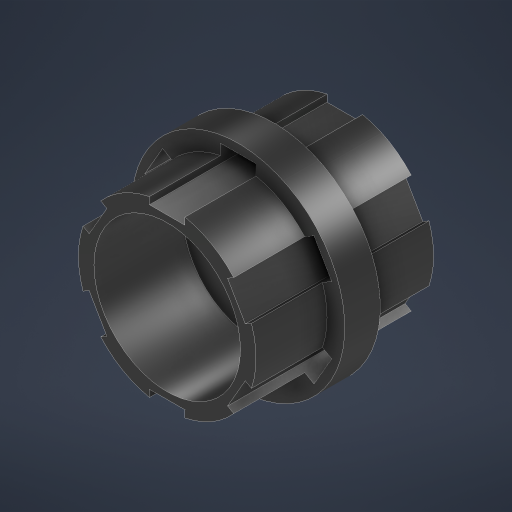
# Autodesk Inventor part: koło
Saved by Autodesk Inventor 2023.4 (Build 274418000, 418)
## iProperties
Created: 2025-10-31
Part Number: koło
Material: Tworzywo sztuczne PET
Document SubType Name: Modeling
Designer: Jakub Borsukiewicz
Density: 1.541 g/cm^3
Appearance: Lśniąca — czarna
Author: Jakub Borsukiewicz
Autodesk Inventor part; units mm, degrees
ref_plane "YZ Plane" through (0, 0, 0) normal (1, 0, 0) x (0, 1, 0)
ref_plane "XZ Plane" through (0, 0, 0) normal (0, 1, 0) x (-1, 0, 0)
sketch "Szkic1" plane through (0, 0, 0) normal (0, 0, 1) x (1, 0, 0)
  line L0 (-14, 0) -> (14, 0) projected
  line L1 (0, -14) -> (0, 14) projected
  circle A0 centre (0, 0) radius 10
  circle A1 centre (0, 0) radius 1.8
  line L2 (-1.3416, 1.2) -> (1.3416, 1.2)
  dimension "d1" = 20
  dimension "d2" = 3.6
  dimension "d3" = 1.2
  constraints: 2 centre point, 2 coincident, 2 end point, 2 point on circle, 1 perpendicular
  measures "d1" diameter of A0
  measures "d2" diameter of A1
  measures "d3" distance between parallel lines of L0 L2
extrude "Wyciągnięcie proste1" add sketch "Szkic1" along normal blind 20 contours A1 L1 A0 L0 | L0 A0 L1 A1 | L2 L1 A1 | L1 A0 L0 A1 | L1 A1 L0 A0 | L2 A1 L1
ref_plane "Płaszczyzna konstrukcyjna1" through (0, 0, 8) normal (0, 0, -1) x (-1, 0, 0)
sketch "Szkic2" plane through (0, 0, 8) normal (0, 0, -1) x (-1, 0, 0)
  circle A0 centre (0, 0) radius 10 projected
  arc A1 (-1.3416, 1.2) -> (1.3416, 1.2) centre (0, 0) ccw projected
  line L0 (1.3416, 1.2) -> (-1.3416, 1.2) projected
  circle A2 centre (0, 0) radius 12
  dimension "d7" = 24
  constraints: 1 centre point, 1 coincident
  measures "d7" diameter of A2
extrude "Wyciągnięcie proste2" add sketch "Szkic2" against normal blind 4 contours A2
sketch "Szkic3" plane through (0, 0, 0) normal (0, 0, -1) x (-1, 0, 0)
  circle A0 centre (0, 0) radius 10 projected
  arc A1 (-1.3416, 1.2) -> (1.3416, 1.2) centre (0, 0) ccw projected
  line L0 (1.3416, 1.2) -> (-1.3416, 1.2) projected
  circle A2 centre (0, 0) radius 12 projected
  circle A3 centre (0, 0) radius 10 projected
  line L1 (16.8, 0) -> (-16.8, 0) projected
  line L2 (0, -16.8) -> (0, 16.8) projected
  line L3 (2, -11) -> (-2, -11)
  line L4 (-2, -11) -> (-2, -9)
  line L5 (-2, -9) -> (2, -9)
  line L6 (2, -9) -> (2, -11)
  circle A4 centre (0, 0) radius 10 projected
  line L7 (2, -11) -> (-2, -9) construction
  line L8 (-2, -11) -> (2, -9) construction
  point P0 (0, -10)
  dimension "d11" = 4
  dimension "d12" = 2
  constraints: 12 end point, 2 midpoint, 2 parallel, 1 horizontal, 1 perpendicular, 1 point on line, 1 vertical alignment, 1 other
  measures "d11" distance of L4.end L5.end
  measures "d12" distance of L3.end L4.end
extrude "Wyciągnięcie proste3" cut sketch "Szkic3" against normal up to surface (20 mm away) contours L6 L3 L2 A0 | A0 L2 L5 L6 | L2 L3 L4 A0 | A0 L4 L5 L2
pattern_circular "Szyk kołowy1" count 6 over 360 about axis through (0, 0, -10) along (0, 0, 1) of "Wyciągnięcie proste3"
sketch "Szkic4" plane through (0, 0, 20) normal (0, 0, 1) x (1, 0, 0)
  circle A0 centre (0, 0) radius 14
  circle A1 centre (0, 0) radius 8.25
  dimension "d20" = 28
  dimension "d21" = 16.5
  constraints: 2 centre point, 2 coincident
  measures "d20" diameter of A0
  measures "d21" diameter of A1
extrude "Wyciągnięcie proste4" cut sketch "Szkic4" against normal blind 10 contours A1
